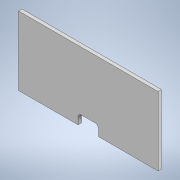
# Autodesk Inventor part: front-panel
Saved by Autodesk Inventor 2021 (Build 250183000, 183)
## iProperties
Created: 2024-06-01
Part Number: front-panel
Material: Generic
Document SubType Name: Modeling
Designer: user
Density: 1 g/cm^3
Appearance: Default
Author: user
Autodesk Inventor part; units mm, degrees
ref_plane "YZ Plane" through (0, 0, 0) normal (1, 0, 0) x (0, 1, 0)
ref_plane "XZ Plane" through (0, 0, 0) normal (0, 1, 0) x (-1, 0, 0)
ref_plane "XY Plane" through (0, 0, 0) normal (0, 0, 1) x (1, 0, 0)
sketch "Sketch1" plane through (0, 0, 0) normal (0, 0, 1) x (1, 0, 0)
  line L0 (-40.3138, 25.1032) -> (45.6862, 25.1032)
  line L1 (45.6862, 25.1032) -> (45.6862, -17.3968)
  line L2 (45.6862, -17.3968) -> (-40.3138, -17.3968)
  line L3 (-40.3138, -17.3968) -> (-40.3138, 25.1032)
  point P0 (0, 0)
  dimension "d0" = 86
  dimension "d1" = 42.5
  constraints: 8 end point, 2 parallel, 1 horizontal, 1 perpendicular
  measures "d0" distance of L0.start L0.end
  measures "d1" distance of L2.end L0.start
extrude "Extrusion1" add sketch "Sketch1" along normal blind 2
sketch "Sketch2" plane through (0, 0, 2) normal (0, 0, 1) x (1, 0, 0)
  line L0 (-40.3138, -17.3968) -> (45.6862, -17.3968) projected
  line L1 (-3.3138, -17.3968) -> (8.6862, -17.3968)
  line L2 (8.6862, -17.3968) -> (8.6862, -11.3968)
  line L3 (8.6862, -11.3968) -> (-3.3138, -11.3968)
  line L4 (-3.3138, -11.3968) -> (-3.3138, -17.3968)
  line L5 (-40.3138, 25.1032) -> (-40.3138, -17.3968) projected
  line L6 (45.6862, -17.3968) -> (45.6862, 25.1032) projected
  point P0 (0, 0)
  dimension "d4" = 6
  dimension "d5" = 12
  dimension "d6" = 37
  dimension "d7" = 86
  constraints: 8 end point, 2 parallel, 1 horizontal, 1 perpendicular, 1 point on line
  measures "d4" distance between parallel lines of L0 L3
  measures "d5" distance of L2.end L3.end
  measures "d6" distance between parallel lines of L5 L4
  measures "d7" distance between parallel lines of L6 L5
extrude "Extrusion2" cut sketch "Sketch2" against normal blind 2
fillet "Fillet1" radius 2 2 edges at (-3.3138, -11.3968, 1) (8.6862, -11.3968, 1)
sketch "Sketch3" plane through (0, 0, 2) normal (0, 0, 1) x (1, 0, 0)
  line L0 (45.6862, 25.1032) -> (-40.3138, 25.1032) projected
  line L1 (45.6862, -17.3968) -> (45.6862, 25.1032) projected
  line L2 (-40.3138, 25.1032) -> (45.6862, 25.1032)
  line L3 (45.6862, 25.1032) -> (45.6862, 23.1032)
  line L4 (45.6862, 23.1032) -> (-40.3138, 23.1032)
  line L5 (-40.3138, 23.1032) -> (-40.3138, 25.1032)
  point P0 (0, 0)
  dimension "d11" = 2
  constraints: 8 end point, 2 parallel, 1 horizontal, 1 perpendicular, 1 point on line
  measures "d11" distance between parallel lines of L4 L0
extrude "Extrusion3" cut sketch "Sketch3" against normal blind 2
sketch "Sketch4" plane through (0, 0, 2) normal (0, 0, 1) x (1, 0, 0)
  line L0 (-40.3138, 23.1032) -> (-40.3138, -17.3968) projected
  line L1 (-40.3138, -17.3968) -> (-3.3138, -17.3968) projected
  line L2 (-40.3138, 23.1032) -> (-38.3138, 23.1032)
  line L3 (-38.3138, 23.1032) -> (-38.3138, -17.3968)
  line L4 (-38.3138, -17.3968) -> (-40.3138, -17.3968)
  line L5 (-40.3138, -17.3968) -> (-40.3138, 23.1032)
  line L6 (8.6862, -17.3968) -> (45.6862, -17.3968) projected
  line L7 (45.6862, 23.1032) -> (43.6862, 23.1032)
  line L8 (43.6862, 23.1032) -> (43.6862, -17.3968)
  line L9 (43.6862, -17.3968) -> (45.6862, -17.3968)
  line L10 (45.6862, -17.3968) -> (45.6862, 23.1032)
  line L11 (45.6862, -17.3968) -> (45.6862, 23.1032) projected
  point P0 (0, 0)
  dimension "d14" = 2
  dimension "d15" = 2
  constraints: 16 end point, 4 parallel, 3 point on line, 2 horizontal, 2 perpendicular, 1 collinear
  measures "d14" distance between parallel lines of L0 L3
  measures "d15" distance between parallel lines of L10 L8
extrude "Extrusion4" cut sketch "Sketch4" against normal blind 2
body "Solid1"
